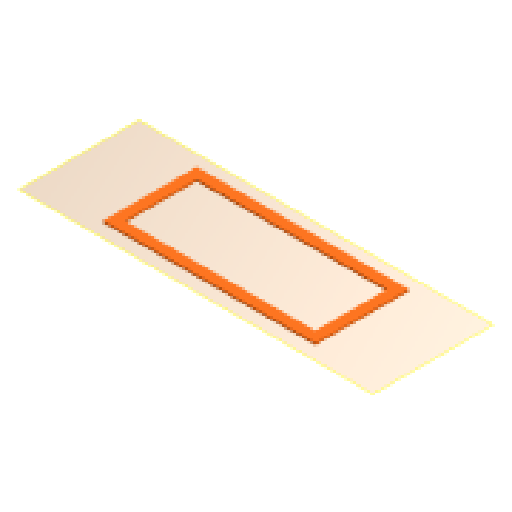
# Autodesk Inventor part: 00_Gasket
Saved by Autodesk Inventor 2024.1 (Build 281209000, 209)
## iProperties
Created: 2024-08-02
Part Number: 00_Gasket
Material: Generisch
Document SubType Name: Modeling
Designer: diederichbenedict
Density: 1 g/cm^3
Appearance: Glatt - Hellorange
Author: diederichbenedict
Autodesk Inventor part; units mm, degrees
ref_plane "YZ Plane" through (0, 0, 0) normal (1, 0, 0) x (0, 1, 0)
ref_plane "XZ Plane" through (0, 0, 0) normal (0, 1, 0) x (-1, 0, 0)
ref_plane "XY Plane" through (0, 0, 0) normal (0, 0, 1) x (1, 0, 0)
ref_plane "Arbeitsebene1" through (0, 0, 0) normal (0, 0, 1) x (1, 0, 0)
sketch "Skizze1" plane through (0, 0, 0) normal (0, 0, 1) x (1, 0, 0)
  circle A0 centre (12, 2.9) radius 1.5 projected
  circle A1 centre (-12, 2.9) radius 1.5 projected
  line L0 (2.5, 12.9) -> (2.5, -7.1) projected
  line L1 (2.5, -7.1) -> (2.25, -7.1) projected
  line L2 (2.25, -7.1) -> (2, -7.1) projected
  line L3 (2, -7.1) -> (1.75, -7.1) projected
  line L4 (1.75, -7.1) -> (1.5, -7.1) projected
  line L5 (1.5, -7.1) -> (1.25, -7.1) projected
  line L6 (1.25, -7.1) -> (1, -7.1) projected
  line L7 (1, -7.1) -> (0.75, -7.1) projected
  line L8 (0.75, -7.1) -> (0.5, -7.1) projected
  line L9 (0.5, -7.1) -> (0.25, -7.1) projected
  line L10 (0.25, -7.1) -> (0, -7.1) projected
  line L11 (0, -7.1) -> (-0.25, -7.1) projected
  line L12 (-0.25, -7.1) -> (-0.5, -7.1) projected
  line L13 (-0.5, -7.1) -> (-0.75, -7.1) projected
  line L14 (-0.75, -7.1) -> (-1, -7.1) projected
  line L15 (-1, -7.1) -> (-1.25, -7.1) projected
  line L16 (-1.25, -7.1) -> (-1.5, -7.1) projected
  line L17 (-1.5, -7.1) -> (-1.75, -7.1) projected
  line L18 (-1.75, -7.1) -> (-2, -7.1) projected
  line L19 (-2, -7.1) -> (-2.25, -7.1) projected
  line L20 (-2.25, -7.1) -> (-2.5, -7.1) projected
  line L21 (-2.5, -7.1) -> (-2.5, 12.9) projected
  line L22 (-2.5, 12.9) -> (-38, 12.9) projected
  line L23 (-38, 12.9) -> (-38, -12.9) projected
  line L24 (-38, -12.9) -> (38, -12.9) projected
  line L25 (38, -12.9) -> (38, 12.9) projected
  line L26 (38, 12.9) -> (2.5, 12.9) projected
  line L27 (35, 11) -> (-35, 11)
  line L28 (-35, 11) -> (-35, -11)
  line L29 (-35, -11) -> (35, -11)
  line L30 (35, -11) -> (35, 11)
  line L31 (35, 11) -> (-35, -11) construction
  line L32 (-35, 11) -> (35, -11) construction
  line L33 (-32.5, 8.5) -> (32.5, 8.5)
  line L34 (32.5, 8.5) -> (32.5, -8.5)
  line L35 (32.5, -8.5) -> (-32.5, -8.5)
  line L36 (-32.5, -8.5) -> (-32.5, 8.5)
  line L37 (-32.5, -8.5) -> (-18.5, -8.5)
  line L38 (-18.5, -8.5) -> (-18.5, 8.5)
  line L39 (-18.5, 8.5) -> (-32.5, 8.5)
  line L40 (-32.5, 8.5) -> (-32.5, -8.5)
  line L41 (32.5, 8.5) -> (18.5, 8.5)
  line L42 (18.5, 8.5) -> (18.5, -8.5)
  line L43 (18.5, -8.5) -> (32.5, -8.5)
  line L44 (32.5, -8.5) -> (32.5, 8.5)
  point P0 (0, 0)
  dimension "d0" = 70
  dimension "d1" = 22
  dimension "d2" = 2.5
  dimension "d5" = 14
  dimension "d6" = 14
  constraints: 36 end point, 8 parallel, 4 perpendicular, 3 horizontal, 2 midpoint, 2 point on line, 3 other
  measures "d0" distance of L29.end L28.end
  measures "d1" distance of L28.end L27.end
  measures "d2" distance between parallel lines of L27 L33
  measures "d5" distance of L39.end L38.end
  measures "d6" distance of L43.end L42.end
extrude "Extrusion1" add sketch "Skizze1" along normal blind 0.5 contours L27 L30 L29 L28 L21 L33 L36 L35 L34 L0 | L0 L33 L21 L27 | L33 L34 L35 L42 | L38 L35 L36 L33
